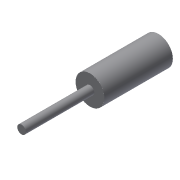
# Autodesk Inventor part: sample pin
Saved by Autodesk Inventor 2015 (Build 190159000, 159)
## iProperties
Created: 2015-01-04
Part Number: sample pin
Material: Generic
Document SubType Name: Modeling
Designer: Peter
Density: 1 g/cm^3
Appearance: Default
Author: Peter
Autodesk Inventor part; units mm, degrees
ref_plane "YZ Plane" through (0, 0, 0) normal (1, 0, 0) x (0, 1, 0)
ref_plane "XZ Plane" through (0, 0, 0) normal (0, 1, 0) x (-1, 0, 0)
ref_plane "XY Plane" through (0, 0, 0) normal (0, 0, 1) x (1, 0, 0)
sketch "Sketch1" plane through (0, 0, 0) normal (0, 0, 1) x (1, 0, 0)
  circle A0 centre (0, 0) radius 5.3479
  constraints: 1 centre point, 1 coincident
extrude "Extrusion1" add sketch "Sketch1" along normal blind 25.4
sketch "Sketch2" plane through (0, 0, 25.4) normal (0, 0, 1) x (1, 0, 0)
  circle A0 centre (0, 0) radius 5.3479 projected
  circle A1 centre (0, 0) radius 1.5875
  dimension "d2" = 3.175
  constraints: 1 centre point, 1 coincident
  measures "d2" diameter of A1
extrude "Extrusion2" add sketch "Sketch2" along normal blind 25.4 contours A1
body "Solid1"
